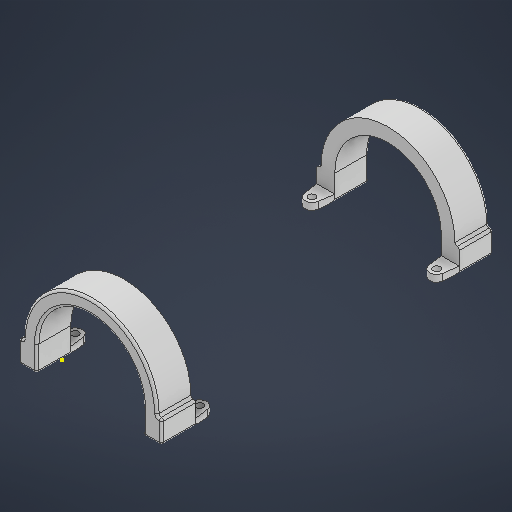
# Autodesk Inventor part: Guardabarros
Saved by Autodesk Inventor 2026.2 (Build 302298000, 298)
## iProperties
Created: 2026-02-04
Part Number: Guardabarros
Material: Generic
Document SubType Name: Modeling
Designer: 06aar
Density: 1 g/cm^3
Appearance: Default
Author: 06aar
Autodesk Inventor part; units mm, degrees
ref_plane "YZ Plane" through (0, 0, 0) normal (1, 0, 0) x (0, 1, 0)
ref_plane "XZ Plane" through (0, 0, 0) normal (0, 1, 0) x (-1, 0, 0)
ref_plane "XY Plane" through (0, 0, 0) normal (0, 0, 1) x (1, 0, 0)
sketch "Sketch3" plane through (0, 0, 0) normal (0, 1, 0) x (-1, 0, 0)
  line L0 (0, 0) -> (7.95, 0)
  line L1 (7.95, 0) -> (7.95, 4)
  line L2 (7.95, 4) -> (0, 4)
  line L3 (0, 4) -> (0, 0)
  circle A0 centre (3.975, -6) radius 1.6
  line L4 (0, 0) -> (0, -9.0302)
  line L5 (3.975, 0) -> (3.975, -6)
  circle A1 centre (3.975, -6) radius 3.1
  line L6 (0, 0) -> (0.9053, -6.432)
  line L7 (7.95, 0) -> (7.0447, -6.432)
  dimension "d1" = 4
  dimension "d2" = 7.95
  dimension "d3" = 3.2
  dimension "d4" = 6
  dimension "d6" = 1.5
  constraints: 17 end point, 2 centre point, 2 parallel, 2 point on circle, 2 tangent, 2 vertical, 1 coincident, 1 horizontal, 1 midpoint, 1 perpendicular
  measures "d1" distance of L0.end L1.end
  measures "d2" distance of L1.end L2.end
  measures "d3" diameter of A0
  measures "d4" distance from line of L0 L5.end
  measures "d6" radial gap between concentric circles of A1 A0
extrude "Extrusion1" add sketch "Sketch3" along normal blind 3 contours L0 L5 A1 L6 | L0 L7 A1 L5 | A1
extrude "Extrusion2" add sketch "Sketch3" along normal blind 10 contours L3 L2 L1 L0
sketch "Sketch4" plane through (0, 3, 0) normal (0, 0, -1) x (-1, 0, 0)
  line L0 (0, 0) -> (0.9053, 0) projected
  line L1 (0, 0) -> (-23.5, 0)
  line L2 (-23.5, 0) -> (-23.5, 8)
  arc A0 (-3.0061, 0) -> (-45.5, 8) centre (-23.5, 8) ccw
  line L3 (0, 0) -> (0, 7) projected
  line L4 (0, 7) -> (7.95, 7) projected
  line L5 (0, 7) -> (0, 0)
  line L6 (2.375, 0) -> (5.575, 0) projected
  line L7 (0, 0) -> (0, 7)
  line L8 (0, 0) -> (2.8106, 0)
  line L9 (4.0031, -3) -> (4, -3)
  line L10 (0, -3) -> (0, 0)
  line L11 (7.95, 7) -> (7.95, -3)
  arc A1 (0, 8) -> (-47, 8) centre (-23.5, 8) ccw
  line L12 (-23.5, 8) -> (0, 8)
  line L13 (2.375, -3) -> (5.575, -3) projected
  line L14 (0, 8) -> (6, 8)
  line L15 (0, -3.0359) -> (0, -3)
  line L16 (-23.5, 8) -> (-53, 8)
  line L17 (-53, 8) -> (-47, 8)
  line L18 (-23.5, 8) -> (-23.5, 37.5)
  arc A2 (6, 8) -> (-53, 8) centre (-23.5, 8) ccw
  line L19 (4.0031, 0) -> (4, 0)
  line L20 (2.8106, 0) -> (0, 0)
  line L21 (0, -3) -> (6, -3)
  line L22 (6, -3) -> (6, 8)
  line L23 (6, 8) -> (0, 8)
  line L24 (0, 8) -> (0, -3)
  point P0 (0, -3)
  point P1 (0, 2.4821)
  point P2 (0, 0)
  point P3 (-23.5, 31.5)
  point P4 (-23.5, 4)
  point P5 (-47, 8)
  point P6 (5, -3)
  point P7 (-23.5, 8)
  point P8 (6, 7)
  point P9 (-23.5, 8)
  dimension "d12" = 90
  dimension "d13" = 8
  dimension "d14" = 44
  dimension "d42" = 90
  dimension "d44" = 6
  dimension "d45" = 23.5
  constraints: 40 end point, 7 point on circle, 6 horizontal, 6 point on line, 3 centre point, 3 coincident, 3 collinear, 3 parallel, 2 perpendicular, 1 midpoint, 1 tangent, 1 vertical
  measures "d12" angle of L2 L1
  measures "d13" distance of L1.end L2.end
  measures "d14" diameter of A0
  measures "d42" angle of L16 L18
  measures "d44" radial gap between concentric circles of A2 A1
  measures "d45" distance from line of point (-23.5, 4) L3
extrude "Extrusion3" add sketch "Sketch4" against normal blind 15 contours L3 L4 L22 L21 L13 L9 L10 | L24 L14 L22 L4 | A1 L18 A2 L14
sketch "Sketch5" plane through (-7.95, 0, 4) normal (0, 0, 1) x (1, 0, 0)
  point P0 (7.95, 0)
ref_plane "Work Plane4" through (23.5, 37.5, 0) normal (1, 0, 0) x (0, 0, -1)
sketch "Sketch6" plane through (-7.95, 0, 4) normal (0, 0, 1) x (1, 0, 0)
  line L0 (1.95, 10) -> (0, 10) projected
  line L1 (0, 0) -> (0, 3) projected
  line L2 (1.95, 10) -> (0, 10)
  line L3 (0, 10) -> (0, 0)
  line L4 (0, 0) -> (1.95, 0)
  line L5 (1.95, 0) -> (1.95, 10)
  point P0 (7.95, 0)
  point P1 (3.95, 0)
  constraints: 8 end point, 2 parallel, 1 horizontal, 1 perpendicular
extrude "Extrusion4" add sketch "Sketch6" along normal up to surface (11 mm away)
fillet "Fillet6" radius 1 1 edges at (-7.95, 10, 7.5)
fillet "Fillet8" radius 1 2 edges at (-3.975, 0, 15) (-7.95, 0, 7.5)
fillet "Fillet9" radius 1 4 edges at (6.883, 27.617, 15) (0, 0.2929, 14.7071) (0, 0, 7) (0, 6, 15)
fillet "Fillet11" radius 1 1 edges at (-6, 10, 7.5)
fillet "Fillet12" radius 1 5 edges at (-6.2841, 10.3012, 15) (-7.6659, 9.6982, 15) (-7.95, 5, 15) (-7.6571, 0.2929, 14.7071) (2.6403, 31.8597, 15)
mirror "Mirror2" about plane through (23.5, 37.5, 0) normal (1, 0, 0)
ref_plane "Work Plane5" through (0, 3, -58.2232) normal (0, 0, -1) x (-1, 0, 0)
mirror "Mirror4" about plane through (0, 3, -58.2232) normal (0, 0, -1)
body "Solid1"
